Barrel_v18 (Autodesk Fusion 360 design; units mm, degrees)
Autodesk Fusion 360 part; units mm, degrees
sketch "Barrels" plane through (0, 0, 0) normal (0, 1, 0) x (1, 0, 0)
  circle A0 centre (0, -20) radius 6
  circle A1 centre (0, -20) radius 5.5
  circle A2 centre (0, 0) radius 5.5
  circle A3 centre (0, 0) radius 6
  circle A4 centre (0, 0) radius 5.4
  dimension "d1" = 12
  dimension "d4" = 11
  dimension "d42" = 20
  dimension "d48" = 11
  dimension "d49" = 12
  dimension "d99" = -0.1
  constraint concentric A0 A1
  constraint coincident A2.centre A3.centre
  constraint concentric A2 A3
  measures "d1" diameter of A0
  measures "d4" diameter of A1
  measures "d42" distance of A2.centre A0.centre
  measures "d48" diameter of A2
  measures "d49" diameter of A3
extrude "Barrel Length" add sketch "Barrels" along normal blind 380 contours A0 makes body 1
pattern_circular "Barrel Pattern" count 6 over 360 about axis through (0, 1.75, 0) along (0, 1, 0) of bodies 1 makes body 2 at (20.5758, 253.3333, 4.9598) makes body 3 at (14.5832, 253.3333, -15.3392) makes body 4 at (-5.9925, 253.3333, -20.2991) makes body 5 at (-20.5758, 253.3333, -4.9598) makes body 6 at (-14.5832, 253.3333, 15.3392)
extrude "Extrude15" add sketch "Barrels" along normal blind 324 from surface at 8 separate body contours A3 makes body 7
ref_plane "WorkPlane1" through (0, 10, 20) normal (0, 1, 0) x (1, 0, 0)
sketch "End Cap" plane through (0, 10, 15) normal (0, 1, 0) x (1, 0, 0)
  circle A0 centre (-17.3205, 5) radius 6
  circle A1 centre (0, -5) radius 6
  circle A2 centre (-17.3205, 25) radius 6
  circle A3 centre (0, 35) radius 6
  circle A4 centre (17.3205, 25) radius 6
  circle A5 centre (17.3205, 5) radius 6
  circle A6 centre (0, 15) radius 30
  circle A7 centre (0, 15) radius 27.5
  circle A8 centre (0, 15) radius 6
  circle A9 centre (-17.3205, 5) radius 6.1
  circle A10 centre (0, -5) radius 6.1
  circle A11 centre (17.3205, 5) radius 6.1
  circle A12 centre (0, 15) radius 6.1
  circle A13 centre (17.3205, 25) radius 6.1
  circle A14 centre (-17.3205, 25) radius 6.1
  circle A15 centre (0, 35) radius 6.1
  dimension "d10" = 60
  dimension "d13" = 55
  dimension "d56" = 0.1
  dimension "d57" = 0.1
  dimension "d58" = 0.1
  dimension "d59" = 0.1
  dimension "d60" = 0.1
  dimension "d61" = 0.1
  dimension "d62" = 0.1
  constraint concentric A6 A7
  measures "d10" diameter of A6
  measures "d13" diameter of A7
extrude "Endcap Base" add sketch "End Cap" along normal mid plane 4 separate body contours A6 | A7 makes body 8
extrude "Endcap Side" add sketch "End Cap" against normal blind 8 from surface at -2 separate body contours A6 makes body 9
ref_plane "WorkPlane2" through (0, 75, 0) normal (0, 1, 0) x (0, 0, 1)
ref_plane "WorkPlane3" through (0, 140, 0) normal (0, 1, 0) x (0, 0, 1)
ref_plane "WorkPlane4" through (0, 270, 0) normal (0, 1, 0) x (0, 0, 1)
sketch "Ring 2" plane through (0, 75, 0) normal (0, 1, 0) x (1, 0, 0)
  circle A0 centre (-17.3205, -10) radius 6
  circle A1 centre (-17.3205, 10) radius 6
  circle A2 centre (0, 20) radius 6
  circle A3 centre (17.3205, 10) radius 6
  circle A4 centre (17.3205, -10) radius 6
  circle A5 centre (0, -20) radius 6
  circle A6 centre (0, 0) radius 30
  circle A7 centre (0, 0) radius 6
  circle A8 centre (-17.3205, -10) radius 6.1
  circle A9 centre (0, -20) radius 6.1
  circle A10 centre (0, 0) radius 6.1
  circle A11 centre (-17.3205, 10) radius 6.1
  circle A12 centre (0, 20) radius 6.1
  circle A13 centre (17.3205, 10) radius 6.1
  circle A14 centre (17.3205, -10) radius 6.1
  dimension "d21" = 60
  dimension "d64" = 0.1
  dimension "d65" = 0.1
  dimension "d66" = 0.1
  dimension "d67" = 0.1
  dimension "d68" = 0.1
  dimension "d69" = 0.1
  dimension "d70" = 0.1
  constraint coincident A6.centre A7.centre
  measures "d21" diameter of A6
extrude "Ring 1 (1)" add sketch "Ring 2" along normal blind 5 separate body contours A6 makes body 10
sketch "Ring 1" plane through (0, 140, 0) normal (0, 1, 0) x (1, 0, 0)
  circle A0 centre (-17.3205, -10) radius 6
  circle A1 centre (0, -20) radius 6
  circle A2 centre (17.3205, -10) radius 6
  circle A3 centre (-17.3205, 10) radius 6
  circle A4 centre (0, 20) radius 6
  circle A5 centre (17.3205, 10) radius 6
  circle A6 centre (0, 0) radius 30
  circle A7 centre (0, 0) radius 6
  circle A8 centre (-17.3205, -10) radius 6.1
  circle A9 centre (0, -20) radius 6.1
  circle A10 centre (17.3205, -10) radius 6.1
  circle A11 centre (0, 0) radius 6.1
  circle A12 centre (-17.3205, 10) radius 6.1
  circle A13 centre (17.3205, 10) radius 6.1
  circle A14 centre (0, 20) radius 6.1
  dimension "d24" = 60
  dimension "d71" = 0.1
  dimension "d72" = 0.1
  dimension "d73" = 0.1
  dimension "d74" = 0.1
  dimension "d75" = 0.1
  dimension "d76" = 0.1
  dimension "d77" = 0.1
  constraint coincident A6.centre A7.centre
  measures "d24" diameter of A6
extrude "Ring 2 (1)" add sketch "Ring 1" along normal blind 5 separate body contours A6 makes body 11
sketch "Ring 3" plane through (0, 270, 0) normal (0, 1, 0) x (1, 0, 0)
  circle A0 centre (0, -20) radius 6
  circle A1 centre (-17.3205, -10) radius 6
  circle A2 centre (-17.3205, 10) radius 6
  circle A3 centre (17.3205, -10) radius 6
  circle A4 centre (17.3205, 10) radius 6
  circle A5 centre (0, 20) radius 6
  circle A6 centre (0, 0) radius 30
  circle A7 centre (0, 0) radius 6
  circle A8 centre (-17.3205, -10) radius 6.1
  circle A9 centre (0, -20) radius 6.1
  circle A10 centre (17.3205, -10) radius 6.1
  circle A11 centre (0, 0) radius 6.1
  circle A12 centre (-17.3205, 10) radius 6.1
  circle A13 centre (0, 20) radius 6.1
  circle A14 centre (17.3205, 10) radius 6.1
  dimension "d27" = 60
  dimension "d78" = 0.1
  dimension "d79" = 0.1
  dimension "d80" = 0.1
  dimension "d81" = 0.1
  dimension "d82" = 0.1
  dimension "d83" = 0.1
  dimension "d84" = 0.1
  constraint coincident A6.centre A7.centre
  measures "d27" diameter of A6
extrude "Ring 3 (1)" add sketch "Ring 3" along normal blind 15 separate body contours A6 makes body 12
ref_plane "WorkPlane5" through (0, 350, 0) normal (0, 1, 0) x (0, 0, 1)
sketch "Base" plane through (0, 350, 0) normal (0, 1, 0) x (1, 0, 0)
  circle A0 centre (-17.3205, -10) radius 6
  circle A1 centre (-17.3205, -10) radius 5.5
  circle A2 centre (0, -20) radius 5.5
  circle A3 centre (0, -20) radius 6
  circle A4 centre (17.3205, -10) radius 6
  circle A5 centre (17.3205, -10) radius 5.5
  circle A6 centre (17.3205, 10) radius 6
  circle A7 centre (17.3205, 10) radius 5.5
  circle A8 centre (0, 20) radius 5.5
  circle A9 centre (0, 20) radius 6
  circle A10 centre (-17.3205, 10) radius 5.5
  circle A11 centre (-17.3205, 10) radius 6
  circle A12 centre (0, 0) radius 35
  line L0 (-30, -35) -> (30, -35)
  line L1 (30, -35) -> (30, 35)
  line L2 (30, 35) -> (-30, 35)
  line L3 (-30, 35) -> (-30, -35)
  circle A13 centre (0, 0) radius 6
  circle A14 centre (-17.3205, -10) radius 6.1
  circle A15 centre (0, -20) radius 6.1
  circle A16 centre (0, 0) radius 6.1
  circle A17 centre (17.3205, -10) radius 6.1
  circle A18 centre (17.3205, 10) radius 6.1
  circle A19 centre (-17.3205, 10) radius 6.1
  circle A20 centre (0, 20) radius 6.1
  line L4 (17.3205, -10) -> (0, -20) construction
  line L5 (8.6603, -15) -> (0, 0) construction
  line L6 (17.3205, 10) -> (0, 20) construction
  line L7 (8.6603, 15) -> (0, 0) construction
  line L8 (0, 0) -> (17.5, 30.3109) construction
  line L9 (0, 0) -> (16.9802, -30.6051) construction
  line L10 (14.1143, -31.6234) -> (19.3609, -28.7125)
  line L11 (19.3609, -28.7125) -> (19.846, -29.5869)
  line L12 (19.846, -29.5869) -> (14.5994, -32.4978)
  line L13 (14.5994, -32.4978) -> (14.1143, -31.6234)
  line L14 (14.1143, -31.6234) -> (19.846, -29.5869) construction
  line L15 (19.3609, -28.7125) -> (14.5994, -32.4978) construction
  line L16 (15.1519, 32.2439) -> (20.3481, 29.2439)
  line L17 (20.3481, 29.2439) -> (19.8481, 28.3779)
  line L18 (19.8481, 28.3779) -> (14.6519, 31.3779)
  line L19 (14.6519, 31.3779) -> (15.1519, 32.2439)
  line L20 (15.1519, 32.2439) -> (19.8481, 28.3779) construction
  line L21 (20.3481, 29.2439) -> (14.6519, 31.3779) construction
  point P0 (16.9802, -30.6051)
  point P1 (17.5, 30.3109)
  dimension "d31" = 70
  dimension "d85" = 0.1
  dimension "d86" = 0.1
  dimension "d87" = 0.1
  dimension "d88" = 0.1
  dimension "d89" = 0.1
  dimension "d90" = 0.1
  dimension "d91" = 0.1
  dimension "d103" = 6
  dimension "d104" = 1
  dimension "d105" = 6
  dimension "d106" = 1
  constraint coincident A12.centre A13.centre
  constraint horizontal L0
  constraint vertical L1
  constraint horizontal L2
  constraint vertical L3
  constraint coincident A4.centre A5.centre
  constraint coincident A2.centre A3.centre
  constraint midpoint L4 L5.start
  constraint coincident A6.centre A7.centre
  constraint coincident A8.centre A9.centre
  constraint midpoint L6 L7.start
  constraint coincident A12 P1
  constraint coincident A12 P0
  constraint perpendicular L10 L11
  constraint parallel L10 L12
  constraint parallel L11 L13
  constraint coincident L14 P0
  constraint coincident L15 P0
  constraint coincident P0 L9.end
  constraint perpendicular L9 L10
  constraint perpendicular L16 L17
  constraint parallel L16 L18
  constraint parallel L17 L19
  constraint coincident L20 P1
  constraint coincident L21 P1
  constraint coincident P1 L8.end
  constraint perpendicular L6 L8
  constraint perpendicular L8 L18
  measures "d31" diameter of A12
  measures "d103" distance of L11.end L12.end
  measures "d104" distance of L10.end L11.end
  measures "d105" distance of L17.end L18.end
  measures "d106" distance of L16.end L17.end
extrude "Base (1)" add sketch "Base" along normal mid plane 40 separate body contours A12 L1 L3 L10 L11 L13 L17 L18 L19 | A13 | A16 makes body 13
sketch "Centre Barrel Hole" plane through (0, 330, 0) normal (0, -1, 0) x (1, 0, 0)
  circle A0 centre (-17.3205, 10) radius 6.1
  circle A1 centre (0, 20) radius 6.1
  circle A2 centre (17.3205, -10) radius 6.1
  circle A3 centre (0, -20) radius 6.1
  circle A4 centre (-17.3205, -10) radius 6.1
  circle A5 centre (17.3205, 10) radius 6.1
  arc A6 (20.0337, -28.6993) -> (30, -18.0278) centre (0, 0) ccw
  line L0 (30, -18.0278) -> (30, 18.0278)
  line L1 (-30, 18.0278) -> (-30, -18.0278)
  circle A7 centre (0, 0) radius 6.1
  line L2 (14.8375, -31.6993) -> (14.6519, -31.3779)
  line L3 (14.6519, -31.3779) -> (19.8481, -28.3779)
  line L4 (19.8481, -28.3779) -> (20.0337, -28.6993)
  arc A8 (30, 18.0278) -> (19.541, 29.0371) centre (0, 0) ccw
  line L5 (19.541, 29.0371) -> (19.3609, 28.7125)
  line L6 (19.3609, 28.7125) -> (14.1143, 31.6234)
  line L7 (14.1143, 31.6234) -> (14.2944, 31.9479)
  arc A9 (14.2944, 31.9479) -> (-30, 18.0278) centre (0, 0) ccw
  arc A10 (-30, -18.0278) -> (14.8375, -31.6993) centre (0, 0) ccw
extrude "Centre Barrel Hole (1)" cut sketch "Centre Barrel Hole" against normal blind 10 contours A7 bodies 13
sketch "Base shaft hole" plane through (30, 0, 0) normal (1, 0, 0) x (0, 1, 0)
  line L0 (330, -18.0278) -> (370, -18.0278)
  line L1 (370, -18.0278) -> (370, 18.0278)
  line L2 (330, 18.0278) -> (330, -18.0278)
  line L3 (330, 18.0278) -> (370, -18.0278) construction
  line L4 (370, 18.0278) -> (330, -18.0278) construction
  circle A0 centre (350, 0) radius 2.55
  line L5 (370, 18.0278) -> (330, 18.0278)
  dimension "d36" = 5.1
  constraint coincident L2.start L3.start
  constraint coincident L0.end L1.start
  constraint coincident L1.end L4.start
  constraint coincident L0.start L2.end
  constraint midpoint L3 A0.centre
  measures "d36" diameter of A0
extrude "Base Shaft" cut sketch "Base shaft hole" against normal blind 60 contours A0 bodies 10 6 4 2 11 9 8 12 13 3 5
combine "Combine1" operation add target body 8 tool bodies 9
extrude "Extrude17" add sketch "Barrels" against normal blind 5 from surface at 8 separate body contours A2 | A3 | A4 makes body 14
fillet "Fillet2" radius 5 tangency weight 0.5 1 faces at (-0.9566, 3, 0.2914) on bodies 14
extrude "Extrude18" add sketch "Barrels" along normal blind 1 from surface at 8 separate body contours A4 makes body 15
combine "Combine2" operation add target body 14 tool bodies 15
sketch "Upper Lock Hole" plane through (16.7376, 0, 30.1679) normal (0.485148, 0, 0.874432) x (0, 1, 0)
  line L0 (330, -3) -> (370, -3)
  line L1 (370, -3) -> (370, 3)
  line L2 (370, 3) -> (330, 3)
  line L3 (330, 3) -> (330, -3)
  line L4 (330, 3) -> (370, -3) construction
  line L5 (370, 3) -> (330, -3) construction
  circle A0 centre (350, 0) radius 3
  circle A1 centre (350, 0) radius 1.7
  dimension "d107" = 6
  dimension "d108" = 3.4
  constraint coincident L2.end L3.start
  constraint coincident L0.end L1.start
  constraint coincident L1.end L2.start
  constraint coincident L0.start L3.end
  constraint midpoint L5 A0.centre
  constraint concentric A0 A1
  measures "d107" diameter of A0
  measures "d108" diameter of A1
extrude "upper lock hole outer" cut sketch "Upper Lock Hole" against normal blind 35 contours A1 bodies 13
extrude "upper lock hole inner" cut sketch "Upper Lock Hole" against normal blind 25 contours A0 bodies 13
sketch "Lock nuts" plane through (0, 370, 0) normal (0, 1, 0) x (-1, 0, 0)
  circle A0 centre (17.3205, -10) radius 6.1
  circle A1 centre (0, -20) radius 6.1
  circle A2 centre (17.3205, 10) radius 6.1
  circle A3 centre (0, 20) radius 6.1
  circle A4 centre (-17.3205, 10) radius 6.1
  circle A5 centre (-17.3205, -10) radius 6.1
  line L0 (-14.6519, -31.3779) -> (-14.8375, -31.6993)
  arc A6 (-14.8375, -31.6993) -> (30, -18.0278) centre (0, 0) ccw
  line L1 (30, -18.0278) -> (30, 18.0278)
  arc A7 (30, 18.0278) -> (-14.2944, 31.9479) centre (0, 0) ccw
  line L2 (-14.2944, 31.9479) -> (-14.1143, 31.6234)
  line L3 (-14.1143, 31.6234) -> (-19.3609, 28.7125)
  line L4 (-19.3609, 28.7125) -> (-19.541, 29.0371)
  arc A8 (-19.541, 29.0371) -> (-30, 18.0278) centre (0, 0) ccw
  line L5 (-30, 18.0278) -> (-30, -18.0278)
  arc A9 (-30, -18.0278) -> (-20.0337, -28.6993) centre (0, 0) ccw
  line L6 (-20.0337, -28.6993) -> (-19.8481, -28.3779)
  line L7 (-19.8481, -28.3779) -> (-14.6519, -31.3779)
  line L8 (-8.6603, 15) -> (0, 0)
  line L9 (0, 0) -> (-2.8868, 5) construction
  line L10 (0, 0) -> (5, 0) construction
  line L11 (-0.7887, 7.366) -> (-5.9848, 4.366)
  line L12 (-5.9848, 4.366) -> (-4.9848, 2.634)
  line L13 (-4.9848, 2.634) -> (0.2113, 5.634)
  line L14 (0.2113, 5.634) -> (-0.7887, 7.366)
  line L15 (-0.7887, 7.366) -> (-4.9848, 2.634) construction
  line L16 (-5.9848, 4.366) -> (0.2113, 5.634) construction
  line L17 (0, 0) -> (-17.5, -30.3109)
  line L18 (0, 0) -> (-2.8868, -5) construction
  line L19 (0, 0) -> (5, 0) construction
  line L20 (-4.9848, -2.634) -> (0.2113, -5.634)
  line L21 (0.2113, -5.634) -> (-0.7887, -7.366)
  line L22 (-0.7887, -7.366) -> (-5.9848, -4.366)
  line L23 (-5.9848, -4.366) -> (-4.9848, -2.634)
  line L24 (-4.9848, -2.634) -> (-0.7887, -7.366) construction
  line L25 (0.2113, -5.634) -> (-5.9848, -4.366) construction
  circle A10 centre (-17.3205, 10) radius 6
  circle A11 centre (0, 20) radius 6
  circle A12 centre (17.3205, 10) radius 6
  circle A13 centre (17.3205, -10) radius 6
  circle A14 centre (0, -20) radius 6
  circle A15 centre (-17.3205, -10) radius 6
  circle A16 centre (0, 20) radius 8
  circle A17 centre (-17.3205, 10) radius 8
  circle A18 centre (-17.3205, -10) radius 8
  circle A19 centre (17.3205, 10) radius 8
  circle A20 centre (17.3205, -10) radius 8
  circle A21 centre (0, -20) radius 8
  point P0 (-2.8868, 5)
  point P1 (-2.8868, -5)
  dimension "d115" = 6
  dimension "d116" = 2
  dimension "d119" = 6
  dimension "d120" = 2
  dimension "d123" = 5
  dimension "d124" = 5
  dimension "d131" = 16
  dimension "d132" = 16
  dimension "d133" = 16
  dimension "d134" = 16
  dimension "d135" = 16
  dimension "d136" = 16
  constraint horizontal L10
  constraint coincident A6.centre A7.centre
  constraint perpendicular L11 L12
  constraint parallel L11 L13
  constraint parallel L12 L14
  constraint coincident L15 P0
  constraint coincident L16 P0
  constraint coincident P0 L9.end
  constraint horizontal L19
  constraint perpendicular L20 L21
  constraint parallel L20 L22
  constraint parallel L21 L23
  constraint coincident L24 P1
  constraint coincident L25 P1
  constraint coincident P1 L18.end
  constraint concentric A11 A16
  constraint concentric A10 A17
  constraint concentric A15 A18
  constraint concentric A12 A19
  constraint concentric A13 A20
  constraint concentric A14 A21
  measures "d115" distance of L12.end L13.end
  measures "d116" distance of L11.end L12.end
  measures "d119" distance of L21.end L22.end
  measures "d120" distance of L20.end L21.end
  measures "d123" vertical distance of A6.centre P0
  measures "d124" vertical distance of A6.centre P1
  measures "d131" diameter of A16
  measures "d132" diameter of A17
  measures "d133" diameter of A18
  measures "d134" diameter of A19
  measures "d135" diameter of A20
  measures "d136" diameter of A21
extrude "lock nuts" cut sketch "Lock nuts" against normal blind 24 contours L8 L11 L13 L14 | L8 L11 L12 L13 | L17 L20 L21 L22 | L17 L20 L22 L23 bodies 13
sketch "Lower Lock Hole" plane through (17.25, 0, -29.8779) normal (0.5, 0, -0.866025) x (0, 1, 0)
  line L0 (330, -3) -> (370, -3)
  line L1 (370, -3) -> (370, 3)
  line L2 (370, 3) -> (330, 3)
  line L3 (330, 3) -> (330, -3)
  line L4 (330, 3) -> (370, -3) construction
  line L5 (370, 3) -> (330, -3) construction
  circle A0 centre (350, 0) radius 3
  circle A1 centre (350, 0) radius 1.7
  dimension "d125" = 6
  dimension "d126" = 3.4
  constraint coincident L2.end L3.start
  constraint coincident L0.end L1.start
  constraint coincident L1.end L2.start
  constraint coincident L0.start L3.end
  constraint midpoint L5 A0.centre
  constraint concentric A0 A1
  measures "d125" diameter of A0
  measures "d126" diameter of A1
extrude "lower lock hole inner" cut sketch "Lower Lock Hole" against normal blind 35 contours A1 bodies 13
extrude "lower lock hole outer" cut sketch "Lower Lock Hole" against normal blind 25 contours A0 bodies 13
extrude "Extrude24" cut sketch "Lock nuts" against normal blind 8 contours A16 | A17 | A18 | A19 | A20 | A21 bodies 13
named bodies: "End Cap", "Ring 1", "Ring 2", "Ring 3", "Base", "Center End Cap"
